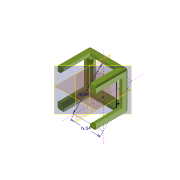
# Autodesk Inventor part: 10_Cube_1x1_v3
Saved by Autodesk Inventor 2022 (Build 260153000, 153)
## iProperties
Created: 2019-07-01
Part Number: 10_Cube_1x1_v3
Material: Generic
Document SubType Name: Modeling
Designer: diederichbenedict
Density: 1 g/cm^3
Appearance: IPHT_Grün
Author: diederichbenedict
Autodesk Inventor part; units mm, degrees
ref_plane "YZ Plane" through (0, 0, 0) normal (1, 0, 0) x (0, 1, 0)
ref_plane "XZ Plane" through (0, 0, 0) normal (0, 1, 0) x (-1, 0, 0)
ref_plane "XY Plane" through (0, 0, 0) normal (0, 0, 1) x (1, 0, 0)
sketch "Sketch1" plane through (0, 0, 0) normal (0, 0, 1) x (1, 0, 0)
  line L0 (-24.9, 24.9) -> (24.9, 24.9)
  line L1 (24.9, 24.9) -> (24.9, -24.9)
  line L2 (24.9, -24.9) -> (-24.9, -24.9)
  line L3 (-24.9, -24.9) -> (-24.9, 24.9)
  line L4 (-24.9, 24.9) -> (24.9, -24.9) construction
  line L5 (24.9, 24.9) -> (-24.9, -24.9) construction
  line L6 (17.05, 17.05) -> (-17.05, 17.05)
  line L7 (-17.05, 17.05) -> (-17.05, -17.05)
  line L8 (-17.05, -17.05) -> (17.05, -17.05)
  line L9 (17.05, -17.05) -> (17.05, 17.05)
  point P0 (0, 0)
  dimension "d0" = 49.8
  dimension "d1" = 49.8
  dimension "d2" = 7.85
  constraints: 20 end point, 4 parallel, 2 midpoint, 2 perpendicular, 1 horizontal, 3 other
  measures "d0" distance of L1.end L2.end
  measures "d1" distance of L0.end L1.end
  measures "d2" distance between parallel lines of L0 L6
extrude "Extrusion1" add sketch "Sketch1" along normal blind 7.7
sketch "Sketch2" plane through (0, 0, 7.7) normal (0, 0, 1) x (1, 0, 0)
  line L0 (17.05, 17.05) -> (17.05, -17.05) projected
  line L1 (17.05, -17.05) -> (-17.05, -17.05) projected
  line L2 (-17.05, -17.05) -> (-17.05, 17.05) projected
  line L3 (-17.05, 17.05) -> (17.05, 17.05) projected
  line L4 (24.9, 24.9) -> (-24.9, 24.9) projected
  line L5 (-24.9, 24.9) -> (-24.9, -24.9) projected
  line L6 (-24.9, -24.9) -> (24.9, -24.9) projected
  line L7 (24.9, -24.9) -> (24.9, 24.9) projected
  line L8 (17.05, -17.05) -> (24.9, -17.05)
  line L9 (24.9, -17.05) -> (24.9, -24.9)
  line L10 (24.9, -24.9) -> (17.05, -24.9)
  line L11 (17.05, -24.9) -> (17.05, -17.05)
  line L12 (17.05, 17.05) -> (-17.05, 17.05) projected
  line L13 (24.9, 24.9) -> (17.05, 24.9)
  line L14 (17.05, 24.9) -> (17.05, 17.05)
  line L15 (17.05, 17.05) -> (24.9, 17.05)
  line L16 (24.9, 17.05) -> (24.9, 24.9)
  line L17 (-24.9, -24.9) -> (-17.05, -24.9)
  line L18 (-17.05, -24.9) -> (-17.05, -17.05)
  line L19 (-17.05, -17.05) -> (-24.9, -17.05)
  line L20 (-24.9, -17.05) -> (-24.9, -24.9)
  line L21 (-24.9, 24.9) -> (-17.05, 24.9)
  line L22 (-17.05, 24.9) -> (-17.05, 17.05)
  line L23 (-17.05, 17.05) -> (-24.9, 17.05)
  line L24 (-24.9, 17.05) -> (-24.9, 24.9)
  point P0 (0, 0)
  constraints: 32 end point, 8 parallel, 4 horizontal, 4 perpendicular
extrude "Extrusion2" add sketch "Sketch2" along normal blind 34.4 contours L14 L4 L7 L15 | L8 L7 L6 L11 | L23 L5 L4 L22 | L18 L6 L5 L19
sketch "Sketch3" plane through (0, 0, 0) normal (0, 0, -1) x (-1, 0, 0)
  line L0 (24.9, -24.9) -> (24.9, 24.9) construction
  line L1 (24.9, 24.9) -> (-24.9, 24.9) construction
  line L2 (-24.9, -24.9) -> (24.9, -24.9) construction
  line L3 (-24.9, 24.9) -> (-24.9, -24.9) construction
  point P0 (20, 20)
  point P1 (20, -20)
  point P2 (-20, -20)
  point P3 (-20, 20)
  dimension "d_1" = 4.9
  dimension "d96" = 4.9
  dimension "d97" = 4.9
  dimension "d98" = 4.9
  dimension "d99" = 4.9
  dimension "d100" = 4.9
  dimension "d101" = 4.9
  dimension "d102" = 4.9
  measures "d_1" distance from line of L1 point (20, 20)
  measures "d96" distance from line of point (20, 20) L0
  measures "d97" distance from line of point (20, -20) L0
  measures "d98" distance from line of point (20, -20) L2
  measures "d99" distance from line of point (-20, -20) L2
  measures "d100" distance from line of point (-20, -20) L3
  measures "d101" distance from line of point (-20, 20) L3
  measures "d102" distance from line of point (-20, 20) L1
hole "Hole1" at (-20, 20, 0) at (-20, -20, 0) at (20, -20, 0) at (20, 20, 0) direction (0, 0, 1) diameter 2.8 depth 16 counterbore diameter 5.5 counterbore depth 3.1
fillet "Fillet1" radius 2 8 edges at (24.9, 24.9, 21.05) (24.9, -24.9, 21.05) (-24.9, -24.9, 21.05) (-24.9, 24.9, 21.05) (-24.9, 0, 0) (0, -24.9, 0) (24.9, 0, 0) (0, 24.9, 0)
sketch "Sketch6" plane through (0, 0, 42.1) normal (0, 0, 1) x (1, 0, 0)
  arc A0 (-22.9, 24.9) -> (-24.9, 22.9) centre (-22.9, 22.9) ccw projected
  line L0 (-24.9, 22.9) -> (-24.9, 17.05) projected
  line L1 (-24.9, 17.05) -> (-17.05, 17.05) projected
  line L2 (-17.05, 17.05) -> (-17.05, 24.9) projected
  line L3 (-17.05, 24.9) -> (-22.9, 24.9) projected
  arc A1 (24.9, 22.9) -> (22.9, 24.9) centre (22.9, 22.9) ccw projected
  line L4 (22.9, 24.9) -> (17.05, 24.9) projected
  line L5 (17.05, 24.9) -> (17.05, 17.05) projected
  line L6 (17.05, 17.05) -> (24.9, 17.05) projected
  line L7 (24.9, 17.05) -> (24.9, 22.9) projected
  arc A2 (22.9, -24.9) -> (24.9, -22.9) centre (22.9, -22.9) ccw projected
  line L8 (24.9, -22.9) -> (24.9, -17.05) projected
  line L9 (24.9, -17.05) -> (17.05, -17.05) projected
  line L10 (17.05, -17.05) -> (17.05, -24.9) projected
  line L11 (17.05, -24.9) -> (22.9, -24.9) projected
  arc A3 (-24.9, -22.9) -> (-22.9, -24.9) centre (-22.9, -22.9) ccw projected
  line L12 (-22.9, -24.9) -> (-17.05, -24.9) projected
  line L13 (-17.05, -24.9) -> (-17.05, -17.05) projected
  line L14 (-17.05, -17.05) -> (-24.9, -17.05) projected
  line L15 (-24.9, -17.05) -> (-24.9, -22.9) projected
  line L16 (0, 38.1838) -> (54, 38.1838) construction
  line L17 (21.1338, 17.05) -> (17.05, 21.1338)
  line L18 (17.05, 24.9) -> (17.05, 17.05) projected
  line L19 (17.05, 21.1338) -> (17.05, 17.05)
  line L20 (17.05, 17.05) -> (21.1338, 17.05)
  line L21 (-17.05, 24.9) -> (-17.05, 17.05) projected
  line L22 (-17.05, 17.05) -> (-17.05, 21.1338)
  line L23 (-17.05, 21.1338) -> (-21.1338, 17.05)
  line L24 (-17.05, 21.1338) -> (-11.2747, 21.1338) construction
  line L25 (-17.05, -17.05) -> (-17.05, 17.05) projected
  line L26 (-21.1338, 17.05) -> (-17.05, 17.05)
  line L27 (-17.05, 17.05) -> (-21.1338, 17.05)
  line L28 (17.05, -17.05) -> (17.05, -24.9) projected
  line L29 (17.05, -17.05) -> (21.1338, -17.05)
  line L30 (24.9, -17.05) -> (17.05, -17.05) projected
  line L31 (21.1338, -17.05) -> (17.05, -21.1338)
  line L32 (17.05, -17.05) -> (17.05, -21.1338)
  line L33 (-17.05, -17.05) -> (-21.1338, -17.05)
  line L34 (-17.05, -17.05) -> (-17.05, -24.9) projected
  line L35 (-17.05, -17.05) -> (-17.05, -21.1338)
  line L36 (-21.1338, -17.05) -> (-17.05, -21.1338)
  line L37 (22.9, 22.9) -> (24.9, 22.9) construction
  line L38 (-22.9, -22.9) -> (22.9, 22.9) construction
  line L39 (-22.9, -22.9) -> (22.9, -22.9) construction
  line L40 (22.9, 22.9) -> (-22.9, 22.9) construction
  line L41 (22.9, -22.9) -> (-22.9, 22.9) construction
  dimension "d111" = 0
  dimension "d120" = 54
  dimension "d121" = 54
  constraints: 34 end point, 9 point on line, 3 collinear, 3 perpendicular, 2 horizontal, 1 equal length, 1 parallel, 1 vertical, 1 other
  measures "d111" vertical distance of L35.end L31.end
  measures "d120" distance between parallel lines of L31 L23
  measures "d121" distance between parallel lines of L36 L17
extrude "Extrusion3" cut sketch "Sketch6" against normal up to surface (34.4 mm away) contours L13 L36 L14 | L2 L1 L23 | L6 L5 L17 | L10 L9 L31
sketch "Sketch7" plane through (-24.9, 17.05, 7.7) normal (0, -1, 0) x (1, 0, 0)
  line L0 (41.95, 0) -> (49.95, 0) construction
  line L1 (41.95, -7.7) -> (41.95, 0) construction
  line L2 (7.85, -7.7) -> (7.85, 0) construction
  line L3 (-0.15, 0) -> (7.85, 0) construction
  line L4 (41.9235, 33.7204) -> (41.95, 0) construction
  line L5 (7.85, 0) -> (7.8764, 33.5861) construction
  line L6 (41.95, 0) -> (7.85, 0) construction
  circle A0 centre (24.9, 17.0366) radius 17.0366 construction
  line L7 (24.9, 55.2203) -> (-13.2838, 17.0366) construction
  line L8 (-13.2838, 17.0366) -> (24.9, -21.1472) construction
  line L9 (24.9, -21.1472) -> (63.0838, 17.0366) construction
  line L10 (63.0838, 17.0366) -> (24.9, 55.2203) construction
  line L11 (24.9, 55.2203) -> (24.9, -21.1472) construction
  line L12 (-13.2838, 17.0366) -> (63.0838, 17.0366) construction
  line L13 (24.9, 55.2203) -> (78.9, 55.2203) construction
  line L14 (46.1838, 0) -> (41.95, 0)
  line L15 (46.1838, 0) -> (41.95, -4.0972)
  line L16 (41.95, 0) -> (41.9235, 33.7204)
  line L17 (41.95, 0) -> (41.95, -4.0972)
  line L18 (46.1838, 0) -> (41.95, 0)
  line L19 (41.95, 0) -> (46.1838, 0)
  line L20 (7.85, 0) -> (3.6162, 0)
  line L21 (3.6162, 0) -> (7.85, -4.0972)
  line L22 (7.85, -4.0972) -> (7.85, 0)
  line L23 (24.9, -36.4773) -> (24.9, 70.8333) projected
  point P0 (44.386, 0)
  point P1 (43.5978, 0)
  point P2 (24.9, 17.0366)
  dimension "d37" = 54
  dimension "d38" = 135
  dimension "d39" = 54
  constraints: 40 end point, 5 point on line, 3 collinear, 3 midpoint, 3 tangent, 2 horizontal, 2 parallel, 1 centre point, 1 equal length, 1 perpendicular, 1 vertical, 1 other
  measures "d37" distance of L7.start L7.end
  measures "d38" angle of L7 L13
  measures "d39" distance of L8.end L7.end
extrude "Extrusion4" cut sketch "Sketch7" along normal up to surface (34.1 mm away)
sketch "Sketch8" plane through (17.05, -24.9, 7.7) normal (-1, 0, 0) x (0, 0, 1)
  line L0 (-4.0838, 41.95) -> (0, 41.95) construction
  line L1 (-4.0838, 7.85) -> (0.1503, 7.85) construction
  line L2 (0.1503, 7.85) -> (0.1503, 3.6159) construction
  line L3 (-4.0838, 7.85) -> (0.1503, 3.6159)
  line L4 (0.1503, 3.6159) -> (0.1503, 7.85)
  line L5 (0.1503, 7.85) -> (-4.0838, 7.85)
  line L6 (-4.0838, 41.95) -> (0, 46.0338)
  line L7 (-4.0838, 41.95) -> (1.6916, 41.95) construction
  line L8 (0.1503, 7.85) -> (0, 41.95)
  line L9 (0, 46.0338) -> (0, 41.95)
  line L10 (0, 41.95) -> (-4.0838, 41.95)
  line L11 (-6, 2) -> (-6, 47.8)
  line L12 (55.2338, 24.9) -> (17.05, 63.0838) construction
  line L13 (17.05, 63.0838) -> (-21.1338, 24.9) construction
  line L14 (-21.1338, 24.9) -> (17.05, -13.2838) construction
  line L15 (17.05, -13.2838) -> (55.2338, 24.9) construction
  line L16 (55.2338, 24.9) -> (-21.1338, 24.9) construction
  line L17 (17.05, 63.0838) -> (17.05, -13.2838) construction
  line L18 (-36.2573, 24.9) -> (70.6573, 24.9) construction
  line L19 (17.05, -28.5573) -> (17.05, 78.3573) construction
  line L20 (0, 41.95) -> (0, 43.5978) construction
  line L21 (0, 7.85) -> (-4.0972, 7.85) construction
  line L22 (-4.0972, 41.95) -> (-4.0972, 7.85) construction
  line L23 (0, 41.95) -> (-4.0972, 41.95) construction
  line L24 (0, 7.85) -> (0, 41.95) construction
  point P0 (-2.4341, 8)
  point P1 (0, 5.414)
  point P2 (17.05, 24.9)
  point P3 (17.05, 24.9)
  point P4 (17.05, 24.9)
  dimension "d122" = 54
  dimension "d123" = 54
  constraints: 32 end point, 5 midpoint, 4 collinear, 3 horizontal, 2 parallel, 2 perpendicular, 2 point on line, 2 vertical, 1 equal length, 6 other
  measures "d122" distance of L12.start L12.end
  measures "d123" distance of L14.end L12.start
extrude "Extrusion5" cut sketch "Sketch8" along normal up to surface (34.1 mm away)
sketch "Sketch9" plane through (0, 0, 42.1) normal (0, 0, 1) x (1, 0, 0)
  arc A0 (19.486, 18.6978) -> (18.6978, 19.486) centre (20, 20) ccw projected
  arc A1 (18.6978, -19.486) -> (19.486, -18.6978) centre (20, -20) ccw projected
  arc A2 (-19.486, -18.6978) -> (-18.6978, -19.486) centre (-20, -20) ccw projected
  arc A3 (-18.6978, 19.486) -> (-19.486, 18.6978) centre (-20, 20) ccw projected
hole "Hole2" at (20, 20, 42.1) at (-20, 20, 42.1) at (20, -20, 42.1) at (-20, -20, 42.1) direction (0, 0, -1) diameter 2.8 depth 12
sketch "Sketch15" plane through (0, 0, 0) normal (0, 0, -1) x (-1, 0, 0)
  line L0 (-17.05, -17.05) -> (-17.05, 17.05) construction
  line L1 (-17.05, 17.05) -> (17.05, 17.05) construction
  line L2 (17.05, 17.05) -> (17.05, -17.05) construction
  line L3 (17.05, -17.05) -> (-17.05, -17.05) construction
  circle A0 centre (-20, 20) radius 2.75 construction
  circle A1 centre (20, -20) radius 2.75 construction
  circle A2 centre (20, 20) radius 2.75 construction
  circle A3 centre (-20, -20) radius 2.75 construction
  line L4 (-22.9, 22.9) -> (22.9, 22.9) construction
  line L5 (-22.9, -22.9) -> (-22.9, 22.9) construction
  line L6 (22.9, -22.9) -> (-22.9, -22.9) construction
  line L7 (22.9, 22.9) -> (22.9, -22.9) construction
  line L8 (17.05, 21.1338) -> (-17.05, 21.1338) construction
  point P0 (0, 0)
  point P1 (-20.8, -14.5)
  point P2 (-14.5, -20.8)
  point P3 (14.5, -20.8)
  point P4 (20.8, -14.5)
  point P5 (20.8, 14.5)
  point P6 (14.5, 20.8)
  point P7 (-14.5, 20.8)
  point P8 (-20.8, 14.5)
hole "Hole8" [suppressed]
ref_plane "Arbeitsebene2" through (24.9, 0, 0) normal (-0.7071, 0, -0.7071) x (0, 1, 0)
ref_plane "Arbeitsebene3" through (0, -17.05, 7.7) normal (1, 0, 0) x (0, 0, -1)
ref_plane "Work Plane4" through (-17.05, 0, 7.7) normal (0, 1, 0) x (1, 0, 0)
equation "\"d1\" = d0"
equation "\"d96\" = d_1"
equation "\"d97\" = d_1"
equation "\"d98\" = d_1"
equation "\"d99\" = d_1"
equation "\"d100\" = d_1"
equation "\"d101\" = d_1"
equation "\"d102\" = d_1"
equation "\"d121\" = d120"
body "Solid1"
